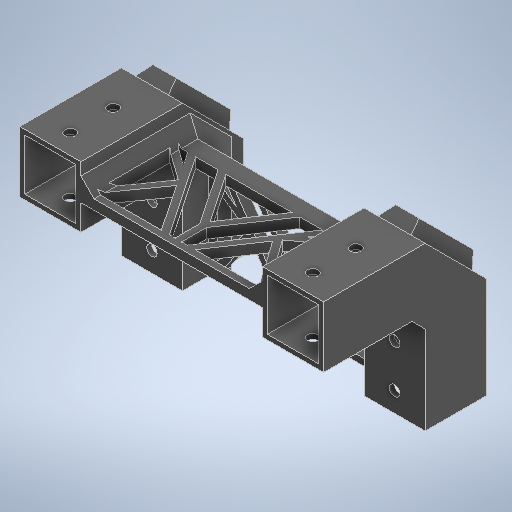
# Autodesk Inventor part: 90_deg
Saved by Autodesk Inventor 2026.1 (Build 301233020, 233B)
## iProperties
Created: 2026-02-01
Part Number: 90_deg
Material: 一般
Document SubType Name: Modeling
Designer: hibik
Density: 1 g/cm^3
Appearance: 既定
Author: hibik
Autodesk Inventor part; units mm, degrees
ref_plane "XZ Plane" through (0, 0, 0) normal (0, 1, 0) x (-1, 0, 0)
ref_plane "XY Plane" through (0, 0, 0) normal (0, 0, 1) x (1, 0, 0)
ref_plane "作業平面1" through (36.75, 0, 0) normal (1, 0, 0) x (0, 1, 0)
sketch "スケッチ1" plane through (0, 0, 0) normal (0, 0, 1) x (1, 0, 0)
  line L0 (36.75, 12.95) -> (36.75, -12.95) projected
  line L1 (29, -7.75) -> (44.5, -7.75)
  line L2 (44.5, -7.75) -> (44.5, 7.75)
  line L3 (44.5, 7.75) -> (29, 7.75)
  line L4 (29, 7.75) -> (29, -7.75)
  line L5 (29, -7.75) -> (44.5, 7.75) construction
  line L6 (44.5, -7.75) -> (29, 7.75) construction
  line L7 (46, -9.25) -> (27.5, -9.25)
  line L8 (27.5, -9.25) -> (27.5, 9.25)
  line L9 (27.5, 9.25) -> (46, 9.25)
  line L10 (46, 9.25) -> (46, -9.25)
  line L11 (46, -9.25) -> (27.5, 9.25) construction
  line L12 (27.5, -9.25) -> (46, 9.25) construction
  point P0 (0, 0)
  point P1 (36.75, 0)
  dimension "d1" = 15.5
  dimension "d2" = 1.5
  constraints: 24 end point, 5 midpoint, 4 parallel, 3 perpendicular, 2 horizontal, 1 horizontal alignment, 1 point on line
  measures "d1" distance of L2.end L3.end
  measures "d2" distance between parallel lines of L9 L3
extrude "押し出し1" add sketch "スケッチ1" along normal blind 40 contours L9 L10 L7 L0 L1 L2 L3 | L0 L3 L4 L1 L7 L8 L9
sketch "スケッチ2" plane through (27.5, 9.25, 0) normal (0, 1, 0) x (1, 0, 0)
  circle A0 centre (9.25, -34) radius 1.6
  line L0 (18.5, -40) -> (0, -40) projected
  circle A1 centre (9.25, -21) radius 1.6
  point P0 (-27.5, 0)
  point P1 (9.25, -40)
  dimension "d5" = 3.2
  dimension "d6" = 6
  dimension "d7" = 3.2
  dimension "d8" = 13
  constraints: 2 centre point, 2 vertical alignment, 1 midpoint
  measures "d5" diameter of A0
  measures "d6" distance from line of L0 A0.centre
  measures "d7" diameter of A1
  measures "d8" distance of A1.centre A0.centre
extrude "押し出し2" cut sketch "スケッチ2" against normal through all
ref_plane "作業平面2" through (27.5, 0, 0) normal (0, 1, 0) x (1, 0, 0)
pattern_circular "円形状パターン1" count 2 over 90 about axis through (27.5, 0, 0) along (1, 0, 0) of "押し出し1", "押し出し2"
sketch "スケッチ3" plane through (46, -9.25, 40) normal (1, 0, 0) x (0, 0, -1)
  line L0 (40, 18.5) -> (0, 18.5) projected
  line L1 (30.75, 18.5) -> (49.25, 0)
  line L2 (40, 9.25) -> (40, 18.5) projected
  line L3 (49.25, 9.25) -> (40, 9.25) projected
  line L4 (49.25, 9.25) -> (49.25, -30.75) projected
  dimension "d14" = 45
  constraints: 2 end point, 2 point on line, 1 midpoint
  measures "d14" angle of L0 L1
extrude "押し出し3" cut sketch "スケッチ3" against normal through all
sketch "スケッチ4" plane through (46, -9.25, 40) normal (1, 0, 0) x (0, 0, -1)
  line L0 (49.25, -2.1213) -> (28.6287, 18.5)
  line L1 (30.75, 18.5) -> (0, 18.5) projected
  line L2 (49.25, 0) -> (30.75, 18.5) projected
  line L3 (49.25, 0) -> (49.25, -30.75) projected
  point P0 (40, 9.25)
  dimension "d17" = 1.5
  constraints: 2 end point, 2 point on line, 1 parallel
  measures "d17" distance between parallel lines of L2 L0
extrude "押し出し4" add sketch "スケッチ4" against normal up to surface (17 mm away)
sketch "スケッチ5" plane through (46, 9.25, 9.25) normal (0, 0.7071068, -0.7071068) x (-1, 0, 0)
  line L0 (4.25, -26.163) -> (14.25, -26.163)
  line L1 (14.25, -26.163) -> (14.25, 0)
  line L2 (14.25, 0) -> (4.25, 0)
  line L3 (4.25, 0) -> (4.25, -26.163)
  line L4 (0, 0) -> (18.5, 0) projected
  line L5 (18.5, -26.163) -> (0, -26.163) projected
  point P0 (46, -13.0815)
  point P1 (9.25, 0)
  point P2 (9.25, -26.163)
  dimension "d20" = 10
  constraints: 8 end point, 4 midpoint, 2 parallel, 1 horizontal, 1 perpendicular, 1 point on line
  measures "d20" distance of L0.start L0.end
extrude "押し出し5" add sketch "スケッチ5" along normal blind 4 draft -20
mirror "ミラー1" about plane through (0, 0, 0) normal (1, 0, 0)
sketch "スケッチ6" plane through (-29, -40, 7.75) normal (-1, 0, 0) x (0, 0, 1)
  line L0 (1.5, 30.75) -> (1.5, 0) projected
  line L1 (1.5, 0) -> (0, 0) projected
  line L2 (0, 30.75) -> (0, 0) projected
  line L3 (-7.75, 30.75) -> (0, 30.75) projected
  line L4 (-7.75, 32.25) -> (-7.75, 30.75) projected
  line L5 (0, 32.25) -> (-7.75, 32.25) projected
  line L6 (0, 40) -> (0, 32.25) projected
  line L7 (1.5, 40) -> (0, 40) projected
  line L8 (1.5, 32.25) -> (1.5, 40) projected
  line L9 (32.25, 32.25) -> (1.5, 32.25) projected
  line L10 (32.25, 47.75) -> (32.25, 32.25) projected
  line L11 (32.25, 49.25) -> (32.25, 47.75) projected
  line L12 (1.5, 49.25) -> (32.25, 49.25) projected
  line L13 (-17, 30.75) -> (1.5, 49.25) projected
  line L14 (-17, 0) -> (-17, 30.75) projected
  line L15 (-15.5, 0) -> (-17, 0) projected
  line L16 (0, 0) -> (-15.5, 0) projected
  line L17 (32.25, 30.75) -> (1.5, 30.75) projected
  line L18 (32.25, 32.25) -> (32.25, 30.75) projected
  line L19 (2.1213, 47.75) -> (32.25, 47.75) projected
  line L20 (2.1213, 47.75) -> (-15.5, 30.1287) projected
  line L21 (-15.5, 30.1287) -> (-15.5, 0) projected
  line L22 (0, 30.75) -> (1.5, 32.25)
  point P0 (-7.75, 40)
  constraints: 2 end point
extrude "押し出し6" cut sketch "スケッチ6" along normal up to surface (15.5 mm away) contours L3 L4 L5 L6 L7 L8 L22
chamfer "面取り1" distance 4 angle 45 1 edges at (-36.75, -9.25, 9.25)
sketch "スケッチ7" plane through (-27.5, -40, -9.25) normal (1, 0, 0) x (0, 0, -1)
  line L0 (-18.5, 49.25) -> (0, 30.75) projected
  line L1 (-18.5, 49.25) -> (-49.25, 49.25) projected
  line L2 (-49.25, 49.25) -> (-49.25, 30.75) projected
  line L3 (-22.5, 30.75) -> (-49.25, 30.75) projected
  line L4 (-18.5, 26.75) -> (-22.5, 30.75) projected
  line L5 (-18.5, 26.75) -> (-18.5, 0) projected
  line L6 (-18.5, 0) -> (0, 0) projected
  line L7 (0, 30.75) -> (0, 0) projected
  line L8 (-49.25, 49.25) -> (-49.25, 30.75) projected
  line L9 (-49.25, 41.5) -> (-17.8211, 41.5)
  line L10 (-17.8211, 41.5) -> (-17.8211, 38.5)
  line L11 (-17.8211, 38.5) -> (-49.25, 38.5)
  line L12 (-49.25, 38.5) -> (-49.25, 41.5)
  line L13 (-10.75, 0) -> (-7.75, 0)
  line L14 (-7.75, 0) -> (-7.75, 31.4289)
  line L15 (-7.75, 31.4289) -> (-10.75, 31.4289)
  line L16 (-10.75, 31.4289) -> (-10.75, 0)
  line L17 (-17.8211, 41.5) -> (-7.75, 31.4289)
  line L18 (-18.5, 49.25) -> (0, 30.75) projected
  line L19 (-21.8921, 38.5) -> (-10.75, 27.3579)
  point P0 (-9.25, 40)
  point P1 (-49.25, 40)
  point P2 (-9.25, 0)
  point P3 (-7.75, 0)
  dimension "d28" = 3
  dimension "d29" = 5
  dimension "d30" = 5
  constraints: 20 end point, 5 parallel, 4 midpoint, 4 point on line, 3 perpendicular, 2 horizontal
  measures "d28" distance between parallel lines of L11 L9
  measures "d29" distance between parallel lines of L0 L17
  measures "d30" distance between parallel lines of L19 L17
extrude "押し出し7" add sketch "スケッチ7" along normal up to surface (55 mm away) contours L9 L10 L11 L2 | L6 L16 L15 L14 | L17 L15 L16 L19 L11 L10
sketch "スケッチ8" plane through (-27.5, 1.5, 40) normal (0, 1, 0) x (1, 0, 0)
  line L0 (27.5, 61.2588) -> (27.5, -10.2098) projected
  line L1 (27.5, 26.4289) -> (17.5, 26.4289)
  line L2 (17.5, 26.4289) -> (27.5, 11.6033)
  line L3 (26.5, 9.5093) -> (26.5, 2)
  line L4 (26.5, 2) -> (24.7923, 2)
  line L5 (24.7923, 2) -> (8.3148, 26.4289)
  line L6 (8.3148, 26.4289) -> (15.0876, 26.4289)
  line L7 (15.0876, 26.4289) -> (26.5, 9.5093)
  line L8 (12.9368, 16) -> (22.3799, 2)
  line L9 (22.3799, 2) -> (3, 2)
  line L10 (3, 2) -> (12.9368, 16)
  line L11 (3, 5.4554) -> (11.7417, 17.7717)
  line L12 (11.7417, 17.7717) -> (3, 23.9764)
  line L13 (3, 23.9764) -> (3, 5.4554)
  line L14 (3, 26.4289) -> (8.5681, 22.4769)
  line L15 (8.5681, 22.4769) -> (5.9024, 26.4289)
  line L16 (5.9024, 26.4289) -> (3, 26.4289)
  line L17 (0, 30.75) -> (0, 0) projected
  line L18 (0, 31.4289) -> (55, 31.4289) projected
  line L19 (0, 0) -> (55, 0) projected
  point P0 (27.5, 40)
  dimension "d33" = 2
  dimension "d34" = 2
  dimension "d35" = 3
  dimension "d36" = 5
  dimension "d37" = 2
  dimension "d38" = 2
  dimension "d39" = 2
  dimension "d40" = 34
  dimension "d41" = 10
  dimension "d42" = 1
  dimension "d43" = 14
  constraints: 32 end point, 10 point on line, 5 parallel, 4 perpendicular, 2 collinear, 1 horizontal, 1 vertical
  measures "d33" distance between parallel lines of L5 L15
  measures "d34" distance between parallel lines of L12 L14
  measures "d35" distance between parallel lines of L17 L13
  measures "d36" distance between parallel lines of L18 L6
  measures "d37" distance between parallel lines of L10 L11
  measures "d38" distance between parallel lines of L2 L7
  measures "d39" distance between parallel lines of L19 L9
  measures "d40" angle of L0 L2
  measures "d41" distance of L1.start L1.end
  measures "d42" distance between parallel lines of L0 L3
  measures "d43" distance from line of L9 L8.start
extrude "押し出し8" cut sketch "スケッチ8" against normal up to surface (3 mm away)
pattern_circular "円形状パターン2" count 2 over 90 about axis through (27.5, 0, 0) along (1, 0, 0) of "押し出し8"
mirror "ミラー2" about plane through (0, 0, 0) normal (1, 0, 0) of "押し出し8", "円形状パターン2", "押し出し6"
chamfer "面取り2" distance 4 angle 45 6 edges at (-27.5, 1.5, 24.2855) (-27.5, -3.5355, 3.5355) (-27.5, -24.2855, -1.5) (27.5, -24.2855, -1.5) (27.5, -3.5355, 3.5355) (27.5, 1.5, 24.2855)
chamfer "面取り3" distance 4 angle 45 1 edges at (36.75, -9.25, 9.25)
equation "\"d5\" = d7"
equation "\"d34\" = d33"
equation "\"d37\" = d33"
equation "\"d38\" = d33"
equation "\"d39\" = d33"
equation "\"d44\" = d37"
